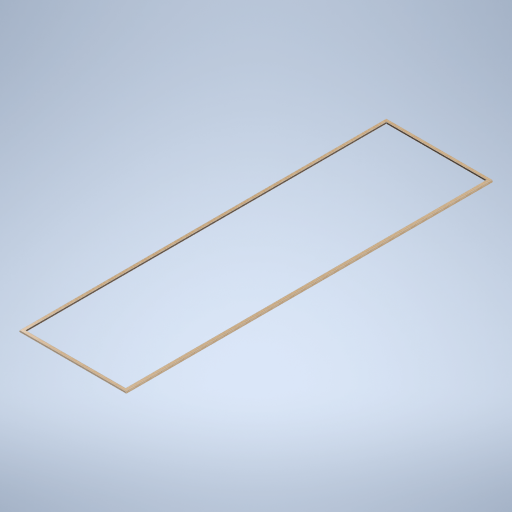
# Autodesk Inventor part: top_wall_frame_MIR
Saved by Autodesk Inventor 2024.2 (Build 282272000, 272)
## iProperties
Created: 2024-05-21
Part Number: top_wall_frame_MIR
Material: Wood (Maple)
Document SubType Name: Modeling
Designer: LOSTER_1
Density: 0.67 g/cm^3
Appearance: Natural Maple - Glossy Dark Tint
Author: LOSTER_1
Autodesk Inventor part; units mm, degrees
ref_plane "YZ Plane" through (0, 0, 0) normal (1, 0, 0) x (0, 1, 0)
ref_plane "XZ Plane" through (0, 0, 0) normal (0, 1, 0) x (-1, 0, 0)
ref_plane "XY Plane" through (0, 0, 0) normal (0, 0, 1) x (1, 0, 0)
sketch "Sketch1" plane through (0, 0, 0) normal (0, 0, 1) x (1, 0, 0)
  line L0 (-4729.3716, 1467.9686) -> (4724.8512, 1467.9686)
  line L1 (-4479.1135, 1609.0039) -> (4474.5931, 1609.0039)
  arc A0 (-4669.1293, 1609.0039) -> (-4729.3716, 1467.9686) centre (3117.1993, -1800.2611) ccw
  arc A1 (4724.8512, 1467.9686) -> (4664.6089, 1609.0039) centre (-3121.7197, -1800.2611) ccw
  line L2 (-4479.1135, 1609.0039) -> (-4669.1293, 1609.0039)
  line L3 (-4479.1135, 1609.0039) -> (-4289.0978, 1609.0039) construction
  line L4 (4474.5931, 1609.0039) -> (4664.6089, 1609.0039)
  point P0 (0, 0)
  constraints: 10 end point, 4 point on circle, 2 centre point, 2 horizontal, 1 collinear
extrude "Extrusion1" add sketch "Sketch1" along normal blind 32302
sketch "Sketch2" plane through (-4669.1293, 1609.0039, 0) normal (0, 1, 0) x (1, 0, 0)
  line L0 (0, 0) -> (0, -32302) projected
  line L1 (9333.7382, 0) -> (0, 0) projected
  line L2 (0, 0) -> (0, -32302) projected
  line L3 (9333.7382, -32302) -> (0, -32302) projected
  line L4 (9333.7382, 0) -> (9333.7382, -32302) projected
  line L5 (9393.9805, 0) -> (9393.9805, -32302) projected
  line L6 (9083.8691, -250) -> (249.8691, -250)
  line L7 (249.8691, -250) -> (249.8691, -32052)
  line L8 (249.8691, -32052) -> (9083.8691, -32052)
  line L9 (9083.8691, -32052) -> (9083.8691, -250)
  line L10 (9083.8691, -250) -> (249.8691, -32052) construction
  line L11 (249.8691, -250) -> (9083.8691, -32052) construction
  point P0 (4669.1293, 0)
  point P1 (4666.8691, -16151)
  dimension "d11" = 8834
  dimension "d12" = 31802
  constraints: 12 end point, 2 midpoint, 2 parallel, 1 horizontal, 1 perpendicular
  measures "d11" distance of L8.end L7.end
  measures "d12" distance of L7.end L6.end
extrude "Extrusion4" cut sketch "Sketch2" against normal through all contours L9 L8 L7 L6
body "Solid1"
